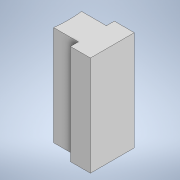
# Autodesk Inventor part: duct_stift
Saved by Autodesk Inventor 2020 (Build 240168000, 168)
## iProperties
Created: 2022-09-28
Part Number: duct_stift
Material: Generisch
Document SubType Name: Modeling
Designer: sp
Density: 1 g/cm^3
Appearance: Vorgabe
Author: sp
Autodesk Inventor part; units mm, degrees
ref_plane "YZ Plane" through (0, 0, 0) normal (1, 0, 0) x (0, 1, 0)
ref_plane "XZ Plane" through (0, 0, 0) normal (0, 1, 0) x (-1, 0, 0)
ref_plane "XY Plane" through (0, 0, 0) normal (0, 0, 1) x (1, 0, 0)
sketch "Skizze1" plane through (0, 0, 0) normal (0, 1, 0) x (-1, 0, 0)
  line L0 (39.5556, 0) -> (-37.1227, 0) construction
  line L1 (0, 37.8779) -> (0, -33.8132) construction
  circle A0 centre (35, 0) radius 30.5
  circle A1 centre (35, 0) radius 29
  line L2 (4.7015, 3.5) -> (0, 3.5)
  line L3 (4.7015, -3.5) -> (0, -3.5)
  line L4 (0, 3.5) -> (0, -3.5)
  line L5 (0, 5.5) -> (-5, 5.5)
  line L6 (-5, 5.5) -> (-5, -5.5)
  line L7 (-5, -5.5) -> (0, -5.5)
  line L8 (0, -5.5) -> (0, 5.5)
  line L9 (4.7015, 3.5) -> (6.212, 3.5)
  line L10 (4.7015, -3.5) -> (6.212, -3.5)
  point P0 (0, 0)
  point P1 (0, 3.5)
  dimension "d0" = 61
  dimension "d1" = 35
  dimension "d2" = 1.5
  dimension "d3" = 7
  dimension "d4" = 5
  dimension "d5" = 11
  constraints: 22 end point, 6 point on line, 4 point on circle, 3 horizontal, 3 perpendicular, 2 centre point, 2 parallel, 1 collinear, 1 vertical, 2 other
  measures "d0" diameter of A0
  measures "d1" distance of point (0, 0) A0.centre
  measures "d2" radial gap between concentric circles of A0 A1
  measures "d3" distance between parallel lines of L3 L2
  measures "d4" distance between parallel lines of L1 L6
  measures "d5" distance of L5.end L6.end
extrude "Extrusion1" add sketch "Skizze1" along normal mid plane 25 contours L9 A1 L10 A0 | A0 L3 L4 L2 | L4 L8 L7 L6 L5 picked at (5.6457, 2.7231)
